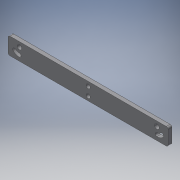
# Autodesk Inventor part: CameraBase
Saved by Autodesk Inventor 2019 (Build 230136000, 136)
## iProperties
Created: 2019-07-15
Part Number: CameraBase
Material: Generic
Document SubType Name: Modeling
Designer: aorfi
Density: 1 g/cm^3
Appearance: Default
Author: aorfi
Autodesk Inventor part; units mm, degrees
ref_plane "YZ Plane" through (0, 0, 0) normal (1, 0, 0) x (0, 1, 0)
ref_plane "XZ Plane" through (0, 0, 0) normal (0, 1, 0) x (-1, 0, 0)
ref_plane "XY Plane" through (0, 0, 0) normal (0, 0, 1) x (1, 0, 0)
sketch "Sketch1" plane through (0, 0, 0) normal (0, 0, 1) x (1, 0, 0)
  line L0 (-85, -9) -> (85, -9)
  line L1 (85, -9) -> (85, 9)
  line L2 (85, 9) -> (-85, 9)
  line L3 (-85, 9) -> (-85, -9)
  line L4 (-85, -9) -> (85, 9) construction
  line L5 (85, -9) -> (-85, 9) construction
  point P0 (0, 0)
  dimension "d3" = 18
  dimension "d26" = 170
  constraints: 12 end point, 2 midpoint, 2 parallel, 1 horizontal, 1 perpendicular
  measures "d3" distance of L2.end L0.start
  measures "d26" distance of L0.start L0.end
extrude "Extrusion1" add sketch "Sketch1" along normal mid plane 4
sketch "Sketch2" plane through (0, 0, -2) normal (0, 0, -1) x (-1, 0, 0)
  circle A0 centre (73, 4) radius 2.5
  arc A1 (79.6458, -2.6458) -> (76.9608, 0.0392) centre (78.3033, -1.3033) ccw
  line L0 (78.3033, -1.3033) -> (73, 4) construction
  line L1 (73, 4) -> (78.3033, 4) construction
  line L2 (78.3033, 4) -> (78.3033, -1.3033) construction
  circle A2 centre (73, 4) radius 7.5 construction
  arc A3 (73, -1.6013) -> (73, -5.3986) centre (73, -3.5) ccw
  arc A4 (73, -5.3986) -> (79.6458, -2.6458) centre (73, 4) ccw
  arc A5 (73, -1.6013) -> (76.9608, 0.0392) centre (73, 4) ccw
  line L3 (85, -9) -> (85, 9) construction
  line L4 (0, -15) -> (0, 15) construction
  circle A6 centre (-73, 4) radius 2.5
  arc A7 (-76.9608, 0.0392) -> (-79.6458, -2.6458) centre (-78.3033, -1.3033) ccw
  arc A8 (-73, -5.3986) -> (-73, -1.6013) centre (-73, -3.5) ccw
  arc A9 (-79.6458, -2.6458) -> (-73, -5.3986) centre (-73, 4) ccw
  arc A10 (-76.9608, 0.0392) -> (-73, -1.6013) centre (-73, 4) ccw
  line L5 (74.0022, 0.0756) -> (77.3469, 3.111) construction
  line L6 (77.3469, 3.111) -> (81.648, 1.7321) construction
  line L7 (81.648, 1.7321) -> (82.6044, -2.6822) construction
  line L8 (82.6044, -2.6822) -> (79.2597, -5.7176) construction
  line L9 (79.2597, -5.7176) -> (74.9586, -4.3387) construction
  line L10 (74.9586, -4.3387) -> (74.0022, 0.0756) construction
  line L11 (85, 9) -> (-85, 9) projected
  point P0 (0, 0)
  point P1 (78.3033, 1.3483)
  point P2 (85, 0)
  dimension "d4" = 5
  dimension "d5" = 3.7973
  dimension "d6" = 45
  dimension "d7" = 3.7973
  dimension "d8" = 15
  dimension "d9" = 12
  dimension "d27" = 7.8232
  dimension "d28" = 5
  constraints: 20 end point, 18 point on circle, 11 centre point, 9 symmetric about line, 6 coincident, 2 midpoint, 2 tangent, 1 horizontal, 1 perpendicular, 1 point on line, 1 vertical, 1 vertical alignment, 18 other
  measures "d4" diameter of A0
  measures "d5" diameter of A1
  measures "d6" angle of L0 L2
  measures "d7" diameter of A3
  measures "d8" diameter of A2
  measures "d9" distance from line of L0.end L3
  measures "d27" distance between parallel lines of L5 L8
  measures "d28" distance from line of L11 L0.end
extrude "Extrusion2" cut sketch "Sketch2" against normal through all
fillet "Fillet1" radius 2 4 edges at (-85, 9, 0) (-85, -9, 0) (85, 9, 0) (85, -9, 0)
sketch "Sketch5" plane through (0, 0, 2) normal (0, 0, 1) x (1, 0, 0)
  line L0 (0, -9) -> (0, 0) construction
  line L1 (0, 0) -> (0, 9) construction
  line L2 (83, 9) -> (-83, 9) construction
  line L3 (-83, -9) -> (83, -9) construction
  point P0 (0, -4.5)
  point P1 (0, 4.5)
  constraints: 4 end point, 4 midpoint, 1 vertical
hole "Hole2" at (0, -4.5, 2) at (0, 4.5, 2) direction (0, 0, -1) diameter 4.496 end through all clearance for "Flat Head Machine Screw (82)" size "#8" standard "Ansi Unified Screw Threads"
equation "\"d7\" = d5"
equation "\"d27\" = d25"
equation "\"d25\" = 7.8232"
body "Solid1"
